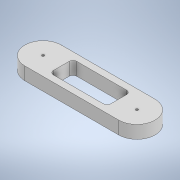
# Autodesk Inventor part: BRAZO BIEN
Saved by Autodesk Inventor 2021 (Build 250183000, 183)
## iProperties
Created: 2023-07-13
Part Number: BRAZO BIEN
Material: Generic
Document SubType Name: Modeling
Designer: PC
Density: 1 g/cm^3
Appearance: Default
Author: PC
Autodesk Inventor part; units mm, degrees
ref_plane "YZ Plane" through (0, 0, 0) normal (1, 0, 0) x (0, 1, 0)
ref_plane "XZ Plane" through (0, 0, 0) normal (0, 1, 0) x (-1, 0, 0)
ref_plane "XY Plane" through (0, 0, 0) normal (0, 0, 1) x (1, 0, 0)
sketch "Sketch1" plane through (0, 0, 0) normal (0, 1, 0) x (-1, 0, 0)
  line L0 (60, -23.199) -> (-60, -23.199)
  line L1 (-60, -23.199) -> (-60, 23.199)
  line L2 (-60, 23.199) -> (60, 23.199)
  line L3 (60, 23.199) -> (60, -23.199)
  line L4 (60, -23.199) -> (-60, 23.199) construction
  line L5 (-60, -23.199) -> (60, 23.199) construction
  point P0 (0, 0)
  dimension "d0" = 120
  dimension "d1" = 46.398
  constraints: 12 end point, 2 midpoint, 2 parallel, 1 horizontal, 1 perpendicular
  measures "d0" distance of L1.end L2.end
  measures "d1" distance of L0.end L1.end
extrude "Extrusion1" add sketch "Sketch1" along normal blind 25
sketch "Sketch2" plane through (0, 25, 0) normal (0, 1, 0) x (1, 0, 0)
  line L0 (60, -23.199) -> (60, 23.199) projected
  circle A0 centre (60, 0) radius 23.199
  line L1 (-60, 23.199) -> (-60, -23.199) projected
  circle A1 centre (-60, 0) radius 23.199
  point P0 (0, 0)
  constraints: 2 midpoint, 2 vertical alignment, 4 other
extrude "Extrusion2" add sketch "Sketch2" against normal blind 25
sketch "Sketch3" plane through (0, 25, 0) normal (0, 1, 0) x (1, 0, 0)
  arc A0 (-60, 23.199) -> (-60, -23.199) centre (-60, 0) ccw projected
  circle A1 centre (-60, 0) radius 17.5
  arc A2 (60, -23.199) -> (60, 23.199) centre (60, 0) ccw projected
  circle A3 centre (60, 0) radius 17.5
  point P0 (0, 0)
  dimension "d6" = 35
  dimension "d7" = 35
  constraints: 2 centre point, 2 coincident
  measures "d6" diameter of A1
  measures "d7" diameter of A3
extrude "Extrusion3" cut sketch "Sketch3" against normal blind 8
sketch "Sketch4" plane through (-60, 17, 0) normal (0, 1, 0) x (1, 0, 0)
  circle A0 centre (0, 0) radius 17.5
  point P0 (60, 0)
  constraints: 1 centre point
extrude "Extrusion4" cut sketch "Sketch4" against normal blind 0.5
sketch "Sketch5" plane through (60, 17, 0) normal (0, 1, 0) x (1, 0, 0)
  circle A0 centre (0, 0) radius 17.5
  point P0 (-60, 0)
  constraints: 1 centre point
extrude "Extrusion5" cut sketch "Sketch5" against normal blind 0.5
sketch "Sketch6" plane through (-60, 16.5, 0) normal (0, 1, 0) x (1, 0, 0)
  circle A0 centre (0, 0) radius 1.55
  circle A1 centre (120, 0) radius 17.5 projected
  circle A2 centre (120, 0) radius 1.55
  point P0 (60, 0)
  dimension "d14" = 3.1
  dimension "d15" = 3.1
  constraints: 2 centre point, 1 coincident
  measures "d14" diameter of A0
  measures "d15" diameter of A2
extrude "Extrusion6" cut sketch "Sketch6" against normal blind 20 contours A0 | A2
sketch "Sketch7" plane through (0, 0, 0) normal (0, -1, 0) x (1, 0, 0)
  circle A0 centre (-60, 0) radius 1.55 projected
  circle A1 centre (-60, 0) radius 10.05
  circle A2 centre (60, 0) radius 1.55 projected
  circle A3 centre (60, 0) radius 10.05
  line L0 (60, 0) -> (53, 0)
  line L1 (60, 0) -> (67, 0)
  circle A4 centre (53, 0) radius 1
  circle A5 centre (67, 0) radius 1
  line L2 (-60, 0) -> (-67, 0)
  line L3 (-60, 0) -> (-53, 0)
  circle A6 centre (-53, 0) radius 1
  circle A7 centre (-67, 0) radius 1
  point P0 (0, 0)
  dimension "d18" = 20.1
  dimension "d19" = 20.1
  dimension "d20" = 7
  dimension "d21" = 7
  dimension "d22" = 2
  dimension "d23" = 2
  dimension "d24" = 7
  dimension "d25" = 7
  dimension "d26" = 2
  dimension "d27" = 2
  constraints: 8 end point, 6 centre point, 6 coincident, 4 horizontal
  measures "d18" diameter of A1
  measures "d19" diameter of A3
  measures "d20" distance of L0.start L0.end
  measures "d21" distance of L0.start L1.end
  measures "d22" diameter of A4
  measures "d23" diameter of A5
  measures "d24" distance of L2.start L2.end
  measures "d25" distance of L2.start L3.end
  measures "d26" diameter of A6
  measures "d27" diameter of A7
extrude "Extrusion7" cut sketch "Sketch7" against normal blind 10.1 contours A4 | A5 | A6 | A7
sketch "Sketch8" plane through (0, 25, 0) normal (0, 1, 0) x (1, 0, 0)
  circle A0 centre (-60, 0) radius 17.5 projected
  circle A1 centre (60, 0) radius 17.5 projected
  line L0 (-60, -17.5) -> (60, -17.5)
  line L1 (60, -17.5) -> (60, 17.5)
  line L2 (60, 17.5) -> (-60, 17.5)
  line L3 (-60, 17.5) -> (-60, -17.5)
  point P0 (0, 0)
  constraints: 8 end point, 2 parallel, 1 horizontal, 1 perpendicular, 4 other
extrude "Extrusion8" cut sketch "Sketch8" against normal blind 8.5 contours A0 L2 A1 L0
sketch "Sketch10" plane through (0, 0, 0) normal (0, -1, 0) x (1, 0, 0)
  point P0 (0, 0)
sketch "Sketch11" plane through (0, 25, 0) normal (0, 1, 0) x (1, 0, 0)
  line L0 (82.2038, 23.199) -> (-84.628, 23.199)
  line L1 (-84.628, 23.199) -> (-84.628, -23.199)
  line L2 (-84.628, -23.199) -> (82.2038, -23.199)
  line L3 (82.2038, -23.199) -> (82.2038, 23.199)
  point P0 (0, 0)
  constraints: 8 end point, 2 parallel, 1 horizontal, 1 perpendicular
extrude "Extrusion9" cut sketch "Sketch11" against normal blind 8.5
sketch "Sketch12" plane through (0, 25, 0) normal (0, 1, 0) x (1, 0, 0)
  line L0 (94.3397, 20.0582) -> (72.0773, 20.0582)
  line L1 (72.0773, 20.0582) -> (72.0773, -24.2462)
  line L2 (72.0773, -24.2462) -> (94.3397, -24.2462)
  line L3 (94.3397, -24.2462) -> (94.3397, 20.0582)
  point P0 (0, 0)
  constraints: 8 end point, 2 parallel, 1 horizontal, 1 perpendicular
extrude "Extrusion10" cut sketch "Sketch12" against normal blind 8.5
sketch "Sketch13" plane through (-60, 16.5, 0) normal (0, 1, 0) x (1, 0, 0)
  circle A0 centre (120, 0) radius 1.55 projected
  line L0 (120, 0) -> (96.801, 0)
  circle A1 centre (0, 0) radius 1.55 projected
  line L1 (0, 0) -> (23.199, 0)
  line L2 (23.199, 0) -> (23.199, -23.199)
  line L3 (120, -23.199) -> (0, -23.199) projected
  line L4 (23.199, 0) -> (23.199, -15)
  line L5 (96.801, 0) -> (96.801, 15)
  line L6 (96.801, 15) -> (23.199, 15)
  line L7 (23.199, 15) -> (23.199, -15)
  line L8 (23.199, -15) -> (96.801, -15)
  line L9 (96.801, -15) -> (96.801, 15)
  point P0 (60, 0)
  dimension "d38" = 23.199
  dimension "d39" = 23.199
  dimension "d40" = 15
  dimension "d41" = 15
  constraints: 18 end point, 3 horizontal, 2 parallel, 2 point on line, 2 vertical, 1 perpendicular
  measures "d38" distance of L0.start L0.end
  measures "d39" distance of L1.start L1.end
  measures "d40" distance of L1.end L4.end
  measures "d41" distance of L0.end L5.end
extrude "Extrusion11" cut sketch "Sketch13" against normal blind 19.75 contours L7 L6 L5 L9 L8 L2
fillet "Fillet3" radius 5 1 edges at (36.801, 8.25, -15)
fillet "Fillet4" radius 5 1 edges at (36.801, 8.25, 15)
fillet "Fillet5" radius 5 1 edges at (-36.801, 8.25, -15)
fillet "Fillet6" radius 5 1 edges at (-36.801, 8.25, 15)
sketch "Sketch14" plane through (0, 0, 0) normal (0, -1, 0) x (1, 0, 0)
  point P0 (0, 0)
body "Solid1"
